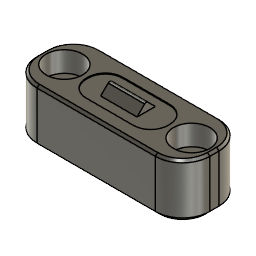
test1 (Autodesk Fusion 360 design; units mm, degrees)
part number: 2026-05-27-10-29-41-988
Autodesk Fusion 360 part; units mm, degrees
note: some values were not read from the file. Chosen so that the rebuilt part matches the saved one: which bodies a step acts on.
sketch "草图1" plane through (0, 0, 0) normal (0, 0, 1) x (1, 0, 0)
  line L0 (-19, -7) -> (19, -7)
  line L1 (19, -7) -> (19, 7)
  line L2 (19, 7) -> (-19, 7)
  line L3 (-19, 7) -> (-19, -7)
  dimension "d1" = 14
  dimension "d2" = 38
  constraint coincident L0.end L1.start
  constraint coincident L0.start L3.end
  constraint coincident L1.end L2.start
  constraint coincident L2.end L3.start
  constraint horizontal L2
  constraint perpendicular L2 L3
  constraint perpendicular L0 L3
  constraint perpendicular L0 L1
  measures "d1" distance of L0.end L2
  measures "d2" distance of L1.end L3
extrude "拉伸1" add sketch "草图1" against normal blind 12 makes body 1
fillet "圆角1" radius 6 4 edges at (19, 7, -6) (-19, 7, -6) (19, -7, -6) (-19, -7, -6) on bodies 1
chamfer "倒角1" distance 1 angle 45 8 edges at (-17.2426, 5.2426, -12) (-19, 0, -12) (-17.2426, -5.2426, -12) (0, -7, -12) (17.2426, -5.2426, -12) (19, 0, -12) (17.2426, 5.2426, -12) (0, 7, -12) measured on face at (-13.2855, 6.9932, -4) measured on face at (4.3333, -2.3333, -12) measured on face at (-13.2855, -6.9932, -4) measured on face at (4.3333, -2.3333, -12) measured on face at (13.2855, -6.9932, -4) measured on face at (4.3333, -2.3333, -12) measured on face at (16.709, 5.7163, -4) measured on face at (4.3333, -2.3333, -12) on bodies 1
sketch "草图2" plane through (0, 0, 0) normal (1, 0, 0) x (0, 0, -1)
  line L0 (0, -2.0071) -> (0, 0)
  line L1 (0, 0) -> (0, 2.0071)
  line L2 (0, 2.0071) -> (-2.0071, 0)
  line L3 (-2.0071, 0) -> (0, -2.0071)
  line L4 (0, 0) -> (0, 100) construction
  constraint coincident L0.end L1.start
  constraint coincident L0.start L3.end
  constraint coincident L1.end L2.start
  constraint coincident L2.end L3.start
  constraint parallel L0 L4
  constraint parallel L1 L4
extrude "拉伸2" add sketch "草图2" along normal blind 4 bodies 1
extrude "拉伸3" add sketch "草图2" against normal blind 4 bodies 1
fillet "圆角2" radius 0.5 1 edges at (0, 0, 2.0071) on bodies 1
sketch "草图3" plane through (0, 0, 0) normal (0, 0, 1) x (1, 0, 0)
  arc A0 (-9, -0.2) -> (-5.2, -4) centre (-5.2, -0.2) ccw
  line L0 (-5.2, -4) -> (5.2, -4)
  arc A1 (5.2, -4) -> (9, -0.2) centre (5.2, -0.2) ccw
  line L1 (9, -0.2) -> (9, 0.2)
  arc A2 (9, 0.2) -> (5.2, 4) centre (5.2, 0.2) ccw
  line L2 (5.2, 4) -> (-5.2, 4)
  arc A3 (-5.2, 4) -> (-9, 0.2) centre (-5.2, 0.2) ccw
  line L3 (-9, 0.2) -> (-9, -0.2)
  point P0 (-7.887, -2.887)
  point P1 (7.887, -2.887)
  point P2 (7.887, 2.887)
  point P3 (-7.887, 2.887)
  dimension "d15" = 3.8
  dimension "d16" = 3.8
  dimension "d17" = 3.8
  dimension "d18" = 3.8
  constraint coincident A0 P0
  constraint coincident A1 P1
  constraint coincident A2 P2
  constraint coincident A3 P3
  constraint coincident A0.end L0.start
  constraint coincident A0.start L3.end
  constraint coincident A1.end L1.start
  constraint coincident L0.end A1.start
  constraint coincident A2.end L2.start
  constraint coincident L1.end A2.start
  constraint coincident A3.end L3.start
  constraint coincident L2.end A3.start
  constraint horizontal L2
  constraint perpendicular L2 L3
  constraint perpendicular L0 L3
  constraint perpendicular L0 L1
  constraint tangent A0 L0
  constraint tangent A0 L3
  constraint tangent L0 A1
  constraint tangent A1 L1
  constraint tangent L1 A2
  constraint tangent A2 L2
  constraint tangent L2 A3
  constraint tangent A3 L3
  measures "d15" radius of A0
  measures "d16" radius of A1
  measures "d17" radius of A2
  measures "d18" radius of A3
extrude "拉伸4" cut sketch "草图3" against normal blind 0.2 bodies 1 makes body 2 at (-1.3333, 0.669, 0)
chamfer "倒角2" distance 0.5 angle 45 8 edges at (-17.2426, 5.2426, 0) (0, 7, 0) (17.2426, 5.2426, 0) (19, 0, 0) (17.2426, -5.2426, 0) (0, -7, 0) (-17.2426, -5.2426, 0) (-19, 0, 0) measured on face at (-13.5703, 6.9728, -3.6667) measured on face at (1.7333, -6, 0) measured on face at (16.4803, 5.8875, -3.6667) measured on face at (1.7333, -6, 0) measured on face at (13.5703, -6.9728, -3.6667) measured on face at (1.7333, -6, 0) measured on face at (-13.5703, -6.9728, -3.6667) measured on face at (1.7333, -6, 0) on bodies 1
sketch "草图4" plane through (0, 0, 0) normal (0, 0, 1) x (1, 0, 0)
  circle A0 centre (-14, 0) radius 4
extrude "拉伸5" cut sketch "草图4" against normal blind 4.5 bodies 1
sketch "草图5" plane through (0, 0, 0) normal (0, 0, 1) x (1, 0, 0)
  circle A0 centre (-14, 0) radius 2.1
extrude "拉伸6" cut sketch "草图5" against normal blind 38 bodies 1
sketch "草图6" plane through (0, 0, 0) normal (0, 0, 1) x (1, 0, 0)
  circle A0 centre (14, 0) radius 4
extrude "拉伸7" cut sketch "草图6" against normal blind 4.5 bodies 1
sketch "草图7" plane through (0, 0, 0) normal (0, 0, 1) x (1, 0, 0)
  circle A0 centre (14, 0) radius 2.1
extrude "拉伸8" cut sketch "草图7" against normal blind 38 bodies 1
